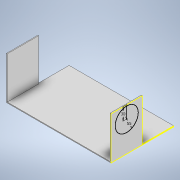
# Autodesk Inventor part: obudowa_elewacji
Saved by Autodesk Inventor 2020 (Build 240168000, 168)
## iProperties
Created: 2020-08-17
Part Number: obudowa_elewacji
Material: Generic
Document SubType Name: Modeling
Designer: Hesekiel
Density: 1 g/cm^3
Appearance: Default
Author: Hesekiel
Autodesk Inventor part; units mm, degrees
ref_plane "YZ Plane" through (0, 0, 0) normal (1, 0, 0) x (0, 1, 0)
ref_plane "XZ Plane" through (0, 0, 0) normal (0, 1, 0) x (-1, 0, 0)
ref_plane "XY Plane" through (0, 0, 0) normal (0, 0, 1) x (1, 0, 0)
sketch "Sketch1" plane through (0, 0, 0) normal (0, 1, 0) x (-1, 0, 0)
  line L0 (-125, 75) -> (125, 75)
  line L1 (125, 75) -> (125, -75)
  line L2 (125, -75) -> (-125, -75)
  line L3 (-125, -75) -> (-125, 75)
  line L4 (-125, 75) -> (125, -75) construction
  line L5 (125, 75) -> (-125, -75) construction
  point P0 (0, 0)
  dimension "d0" = 250
  dimension "d1" = 150
  constraints: 12 end point, 2 midpoint, 2 parallel, 1 horizontal, 1 perpendicular
  measures "d0" distance of L1.end L2.end
  measures "d1" distance of L0.end L1.end
extrude "Extrusion1" add sketch "Sketch1" along normal blind 2
sketch "Sketch2" plane through (0, 2, 0) normal (0, 1, 0) x (1, 0, 0)
  line L0 (-125, 75) -> (-125, -75) projected
  line L1 (-125, -75) -> (-123, -75)
  line L2 (-125, -75) -> (125, -75) projected
  line L3 (-123, -75) -> (-123, 0)
  line L4 (-123, 0) -> (-125, 0)
  line L5 (-125, -75) -> (-125, 0)
  line L6 (125, -75) -> (125, 75) projected
  line L7 (125, -75) -> (123, -75)
  line L8 (123, -75) -> (123, 0)
  line L9 (123, 0) -> (125, 0)
  line L10 (125, -75) -> (125, 0)
  point P0 (0, 0)
  dimension "d4" = 2
  dimension "d5" = 75
  dimension "d8" = 2
  dimension "d9" = 75
  constraints: 16 end point, 2 collinear, 2 midpoint, 2 perpendicular, 2 point on line
  measures "d4" distance of L0.end L1.end
  measures "d5" distance of L1.end L3.end
  measures "d8" distance of L2.end L7.end
  measures "d9" distance of L7.end L8.end
extrude "Extrusion2" add sketch "Sketch2" along normal blind 100
sketch "Sketch3" plane through (125, 0, 75) normal (1, 0, 0) x (0, 0, -1)
  line L0 (0, 0) -> (150, 0) projected
  line L1 (150, 0) -> (150, 2) projected
  line L2 (75, 2) -> (150, 2) projected
  line L3 (75, 2) -> (75, 102) projected
  line L4 (0, 102) -> (75, 102) projected
  line L5 (0, 0) -> (0, 102) projected
  line L6 (0, 102) -> (75, 102) projected
  line L7 (37.5, 102) -> (37.5, 72)
  circle A0 centre (37.5, 72) radius 27.5
  point P0 (75, 0)
  dimension "d12" = 30
  dimension "d13" = 55
  constraints: 2 end point, 1 centre point, 1 coincident, 1 midpoint, 1 vertical
  measures "d12" distance of L7.start L7.end
  measures "d13" diameter of A0
body "Solid1"
